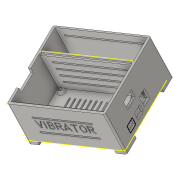
# Autodesk Inventor part: ARDUINO_DUE_CASE_BOTTOM
Saved by Autodesk Inventor 2016 (Build 200138000, 138)
## iProperties
Created: 2015-05-21
Part Number: ARDUINO_DUE_CASE_BOTTOM
Material: Generic
Document SubType Name: Modeling
Designer: Admin
Density: 1 g/cm^3
Appearance: Default
Author: Admin
Autodesk Inventor part; units mm, degrees
ref_plane "YZ Plane" through (0, 0, 0) normal (1, 0, 0) x (0, 1, 0)
ref_plane "XZ Plane" through (0, 0, 0) normal (0, 1, 0) x (-1, 0, 0)
ref_plane "XY Plane" through (0, 0, 0) normal (0, 0, 1) x (1, 0, 0)
sketch "Skizze1" plane through (0, 0, 0) normal (0, 1, 0) x (-1, 0, 0)
  line L0 (0, 0) -> (110, 0)
  line L1 (110, 0) -> (110, 88)
  line L2 (110, 88) -> (0, 88)
  line L3 (0, 88) -> (0, 0)
  dimension "d0" = 110
  dimension "d1" = 88
  constraints: 8 end point, 2 parallel, 1 horizontal, 1 perpendicular
  measures "d0" distance of L2.end L1.end
  measures "d1" distance of L1.end L0.end
extrude "Extrusion1" add sketch "Skizze1" along normal blind 50
sketch "Skizze2" plane through (0, 50, 0) normal (0, 1, 0) x (1, 0, 0)
  line L0 (-3, -5) -> (-107, -5)
  line L1 (-107, -5) -> (-107, -63)
  line L2 (-107, -63) -> (-3, -63)
  line L3 (-3, -63) -> (-3, -5)
  point P0 (0, 0)
  dimension "d4" = 104
  dimension "d5" = 58
  constraints: 8 end point, 2 parallel, 1 horizontal, 1 perpendicular
  measures "d4" distance of L2.end L1.end
  measures "d5" distance of L1.end L0.end
extrude "Extrusion2" cut sketch "Skizze2" against normal blind 47
sketch "Skizze3" plane through (0, 50, 0) normal (0, 1, 0) x (1, 0, 0)
  point P0 (0, 0)
sketch "Skizze6" plane through (0, 3, 0) normal (0, 1, 0) x (1, 0, 0)
  circle A0 centre (-91, -9.5) radius 4.5
  point P0 (0, 0)
  dimension "d16" = 9
  constraints: 1 centre point
  measures "d16" diameter of A0
extrude "Extrusion5" add sketch "Skizze6" along normal blind 4 draft -30
sketch "Skizze7" plane through (0, 3, 0) normal (0, 1, 0) x (1, 0, 0)
  circle A0 centre (-91, -58.5) radius 4.5
  point P0 (0, 0)
  dimension "d19" = 9
  constraints: 1 centre point
  measures "d19" diameter of A0
extrude "Extrusion6" add sketch "Skizze7" along normal blind 4 draft -30
sketch "Skizze8" plane through (-91, 7, 9.5) normal (0, 1, 0) x (1, 0, 0)
  point P0 (91, 9.5)
sketch "Skizze9" plane through (0, 3, 0) normal (0, 1, 0) x (1, 0, 0)
  circle A0 centre (-15.5, -9.5) radius 4.5
  point P0 (0, 0)
  dimension "d22" = 9
  constraints: 1 centre point
  measures "d22" diameter of A0
extrude "Extrusion7" add sketch "Skizze9" along normal blind 4 draft -30
sketch "Skizze10" plane through (0, 3, 0) normal (0, 1, 0) x (1, 0, 0)
  circle A0 centre (-9.5, -58.5) radius 4.5
  point P0 (0, 0)
  dimension "d25" = 9
  constraints: 1 centre point
  measures "d25" diameter of A0
extrude "Extrusion8" add sketch "Skizze10" along normal blind 4 draft -30
sketch "Skizze12" plane through (0, 50, 0) normal (0, 1, 0) x (1, 0, 0)
  line L0 (-3, -5) -> (-3, -63) projected
  line L1 (-3, -5) -> (-107, -5)
  line L2 (-107, -5) -> (-107, -3)
  line L3 (-107, -3) -> (-3, -3)
  line L4 (-3, -3) -> (-3, -5)
  point P0 (0, 0)
  dimension "d32" = 2
  constraints: 8 end point, 2 parallel, 1 horizontal, 1 perpendicular
  measures "d32" distance of L1.end L2.end
extrude "Extrusion10" cut sketch "Skizze12" against normal blind 2
sketch "Skizze13" plane through (0, 3, 0) normal (0, 1, 0) x (1, 0, 0)
  point P0 (0, 0)
sketch "Skizze14" plane through (0, 3, 0) normal (0, 1, 0) x (1, 0, 0)
  point P0 (0, 0)
sketch "Skizze15" plane through (-91, 7, 58.5) normal (0, 1, 0) x (1, 0, 0)
  circle A0 centre (0, 0) radius 1.25
  point P0 (91, 58.5)
  dimension "d35" = 2.5
  constraints: 1 centre point
  measures "d35" diameter of A0
extrude "Extrusion11" cut sketch "Skizze15" against normal blind 10
sketch "Skizze16" plane through (-91, 7, 9.5) normal (0, 1, 0) x (1, 0, 0)
  circle A0 centre (0, 0) radius 1.25
  point P0 (91, 9.5)
  dimension "d38" = 2.5
  constraints: 1 centre point
  measures "d38" diameter of A0
extrude "Extrusion12" cut sketch "Skizze16" against normal blind 10
sketch "Skizze17" plane through (-15.5, 7, 9.5) normal (0, 1, 0) x (1, 0, 0)
  circle A0 centre (0, 0) radius 1.25
  point P0 (15.5, 9.5)
  dimension "d41" = 2.5
  constraints: 1 centre point
  measures "d41" diameter of A0
extrude "Extrusion13" cut sketch "Skizze17" against normal blind 10
sketch "Skizze18" plane through (-9.5, 7, 58.5) normal (0, 1, 0) x (1, 0, 0)
  circle A0 centre (0, 0) radius 1.25
  point P0 (9.5, 58.5)
  dimension "d44" = 2.5
  constraints: 1 centre point
  measures "d44" diameter of A0
extrude "Extrusion14" cut sketch "Skizze18" against normal blind 10
sketch "Skizze29" plane through (0, 0, 0) normal (0, 0, -1) x (-1, 0, 0)
  line L0 (110, 50) -> (0, 50) construction
  line L1 (110, 0) -> (0, 0) construction
  line L2 (0, 50) -> (110, 0) construction
  line L3 (110, 50) -> (0, 0) construction
  line L4 (21.7553, 30.2834) -> (88.2914, 30.2834) construction
  line L5 (88.2914, 30.2834) -> (88.2914, 19.7381) construction
  line L6 (88.2914, 19.7381) -> (21.7553, 19.7381) construction
  line L7 (21.7553, 19.7381) -> (21.7553, 30.2834) construction
  line L8 (29.1209, 29.4232) -> (26.6631, 20.7135)
  spline S0 degree 2 poles (26.6631, 20.7135) (26.5172, 20.1913) (25.8951, 20.1913) knots 0 0 0 1 1 1
  spline S1 degree 2 poles (25.8951, 20.1913) (25.2653, 20.1913) (25.104, 20.6982) knots 0 0 0 1 1 1
  line L9 (25.104, 20.6982) -> (22.3467, 29.4078)
  spline S2 degree 2 poles (22.3467, 29.4078) (22.316, 29.5231) (22.316, 29.6306) knots 0 0 0 1 1 1
  spline S3 degree 2 poles (22.316, 29.6306) (22.316, 29.8764) (22.677, 30.2066) (22.9227, 30.2066) knots 0 0 0 1 2 2 2
  spline S4 degree 2 poles (22.9227, 30.2066) (23.3298, 30.2066) (23.4604, 29.7842) knots 0 0 0 1 1 1
  line L10 (23.4604, 29.7842) -> (25.8874, 22.3264)
  line L11 (25.8874, 22.3264) -> (27.9919, 29.7688)
  spline S5 degree 2 poles (27.9919, 29.7688) (28.1071, 30.2066) (28.5141, 30.2066) knots 0 0 0 1 1 1
  spline S6 degree 2 poles (28.5141, 30.2066) (28.7599, 30.2066) (29.1516, 29.8687) (29.1516, 29.5999) knots 0 0 0 1 2 2 2
  spline S7 degree 2 poles (29.1516, 29.5999) (29.1516, 29.5154) (29.1209, 29.4232) knots 0 0 0 1 1 1
  spline S8 degree 2 poles (32.5771, 20.8441) (32.5771, 20.222) (31.9857, 20.222) knots 0 0 0 1 1 1
  spline S9 degree 2 poles (31.9857, 20.222) (31.3866, 20.222) (31.3866, 20.8441) knots 0 0 0 1 1 1
  line L12 (31.3866, 20.8441) -> (31.3866, 29.5845)
  spline S10 degree 2 poles (31.3866, 29.5845) (31.3866, 30.1913) (31.9857, 30.1913) knots 0 0 0 1 1 1
  spline S11 degree 2 poles (31.9857, 30.1913) (32.5771, 30.1913) (32.5771, 29.5845) knots 0 0 0 1 1 1
  line L13 (32.5771, 29.5845) -> (32.5771, 20.8441)
  spline S12 degree 2 poles (41.8552, 23.1252) (41.8552, 20.3525) (38.7599, 20.3525) knots 0 0 0 1 1 1
  line L14 (38.7599, 20.3525) -> (35.4266, 20.3525)
  line L15 (35.4266, 20.3525) -> (35.4266, 30.2066)
  line L16 (35.4266, 30.2066) -> (38.6293, 30.2066)
  spline S13 degree 2 poles (38.6293, 30.2066) (40.081, 30.2066) (40.9258, 29.4539) knots 0 0 0 1 1 1
  spline S14 degree 2 poles (40.9258, 29.4539) (41.7246, 28.7089) (41.7246, 27.457) knots 0 0 0 1 1 1
  spline S15 degree 2 poles (41.7246, 27.457) (41.7246, 26.2281) (40.7184, 25.3525) knots 0 0 0 1 1 1
  spline S16 degree 2 poles (40.7184, 25.3525) (41.8552, 24.7151) (41.8552, 23.1252) knots 0 0 0 1 1 1
  spline S17 degree 2 poles (40.68, 23.1406) (40.68, 24.7688) (38.6831, 24.7688) knots 0 0 0 1 1 1
  line L17 (38.6831, 24.7688) -> (36.6017, 24.7688)
  line L18 (36.6017, 24.7688) -> (36.6017, 21.5737)
  line L19 (36.6017, 21.5737) -> (38.7599, 21.5737)
  spline S18 degree 2 poles (38.7599, 21.5737) (40.68, 21.5737) (40.68, 23.1406) knots 0 0 0 1 1 1
  spline S19 degree 2 poles (40.5495, 27.4724) (40.5495, 28.202) (39.5126, 28.9854) (38.6293, 28.9854) knots 0 0 0 1 2 2 2
  line L20 (38.6293, 28.9854) -> (36.6017, 28.9854)
  line L21 (36.6017, 28.9854) -> (36.6017, 25.99)
  line L22 (36.6017, 25.99) -> (38.7753, 25.99)
  spline S20 degree 2 poles (38.7753, 25.99) (40.5495, 25.99) (40.5495, 27.4724) knots 0 0 0 1 1 1
  spline S21 degree 2 poles (51.041, 27.3188) (51.041, 25.8057) (50.0502, 25.0453) knots 0 0 0 1 1 1
  spline S22 degree 2 poles (50.0502, 25.0453) (49.3974, 24.5538) (48.7446, 24.5538) knots 0 0 0 1 1 1
  line L23 (48.7446, 24.5538) -> (48.5986, 24.5461)
  line L24 (48.5986, 24.5461) -> (50.9258, 21.2128)
  spline S23 degree 2 poles (50.9258, 21.2128) (51.041, 21.0361) (51.041, 20.8441) knots 0 0 0 1 1 1
  spline S24 degree 2 poles (51.041, 20.8441) (51.041, 20.5983) (50.6647, 20.222) (50.4343, 20.222) knots 0 0 0 1 2 2 2
  spline S25 degree 2 poles (50.4343, 20.222) (50.1578, 20.222) (49.9811, 20.4831) knots 0 0 0 1 1 1
  line L25 (49.9811, 20.4831) -> (47.1163, 24.5538)
  line L26 (47.1163, 24.5538) -> (45.2115, 24.5538)
  line L27 (45.2115, 24.5538) -> (45.2115, 20.8441)
  spline S26 degree 2 poles (45.2115, 20.8441) (45.2115, 20.222) (44.6201, 20.222) knots 0 0 0 1 1 1
  spline S27 degree 2 poles (44.6201, 20.222) (44.0211, 20.222) (44.0211, 20.8441) knots 0 0 0 1 1 1
  line L28 (44.0211, 20.8441) -> (44.0211, 30.1836)
  line L29 (44.0211, 30.1836) -> (48.2223, 30.1836)
  spline S28 degree 2 poles (48.2223, 30.1836) (49.3667, 30.1836) (50.1808, 29.4386) knots 0 0 0 1 1 1
  spline S29 degree 2 poles (50.1808, 29.4386) (51.041, 28.6244) (51.041, 27.3188) knots 0 0 0 1 1 1
  spline S30 degree 2 poles (49.8659, 27.3188) (49.8659, 28.0868) (49.3744, 28.5553) knots 0 0 0 1 1 1
  spline S31 degree 2 poles (49.3744, 28.5553) (48.9058, 28.9777) (48.2223, 28.9777) knots 0 0 0 1 1 1
  line L30 (48.2223, 28.9777) -> (45.2115, 28.9777)
  line L31 (45.2115, 28.9777) -> (45.2115, 25.775)
  line L32 (45.2115, 25.775) -> (48.7446, 25.775)
  spline S32 degree 2 poles (48.7446, 25.775) (49.0671, 25.775) (49.3974, 26.0822) knots 0 0 0 1 1 1
  spline S33 degree 2 poles (49.3974, 26.0822) (49.8659, 26.5046) (49.8659, 27.3188) knots 0 0 0 1 1 1
  spline S34 degree 2 poles (60.5802, 21.0207) (60.6186, 20.8902) (60.6186, 20.775) knots 0 0 0 1 1 1
  spline S35 degree 2 poles (60.6186, 20.775) (60.6186, 20.5292) (60.2422, 20.2066) (60.0118, 20.2066) knots 0 0 0 1 2 2 2
  spline S36 degree 2 poles (60.0118, 20.2066) (59.5971, 20.2066) (59.4512, 20.583) knots 0 0 0 1 1 1
  line L33 (59.4512, 20.583) -> (58.8751, 22.0653)
  line L34 (58.8751, 22.0653) -> (54.1209, 22.0653)
  line L35 (54.1209, 22.0653) -> (53.5525, 20.583)
  spline S37 degree 2 poles (53.5525, 20.583) (53.4066, 20.2066) (53.0149, 20.2066) knots 0 0 0 1 1 1
  spline S38 degree 2 poles (53.0149, 20.2066) (52.7691, 20.2066) (52.3928, 20.5369) (52.3928, 20.775) knots 0 0 0 1 2 2 2
  spline S39 degree 2 poles (52.3928, 20.775) (52.3928, 20.8902) (52.4389, 21.0207) knots 0 0 0 1 1 1
  line L36 (52.4389, 21.0207) -> (55.7184, 29.8149)
  spline S40 degree 2 poles (55.7184, 29.8149) (55.8951, 30.2834) (56.4327, 30.2834) knots 0 0 0 1 1 1
  spline S41 degree 2 poles (56.4327, 30.2834) (56.9857, 30.2834) (57.1624, 29.8149) knots 0 0 0 1 1 1
  line L37 (57.1624, 29.8149) -> (60.5802, 21.0207)
  line L38 (58.422, 23.2865) -> (56.4327, 28.371)
  line L39 (56.4327, 28.371) -> (54.5817, 23.2865)
  line L40 (54.5817, 23.2865) -> (58.422, 23.2865)
  line L41 (68.7522, 28.9086) -> (66.1793, 28.9086)
  line L42 (66.1793, 28.9086) -> (66.1793, 20.3909)
  spline S42 degree 2 poles (66.1793, 20.3909) (66.1793, 19.7381) (65.5571, 19.7381) knots 0 0 0 1 1 1
  spline S43 degree 2 poles (65.5571, 19.7381) (64.9273, 19.7381) (64.9273, 20.3909) knots 0 0 0 1 1 1
  line L43 (64.9273, 20.3909) -> (64.9273, 28.9086)
  line L44 (64.9273, 28.9086) -> (62.3544, 28.9086)
  spline S44 degree 2 poles (62.3544, 28.9086) (61.7169, 28.9086) (61.7169, 29.5538) knots 0 0 0 1 1 1
  spline S45 degree 2 poles (61.7169, 29.5538) (61.7169, 30.1913) (62.3544, 30.1913) knots 0 0 0 1 1 1
  line L45 (62.3544, 30.1913) -> (68.7522, 30.1913)
  spline S46 degree 2 poles (68.7522, 30.1913) (69.3974, 30.1913) (69.3974, 29.5538) knots 0 0 0 1 1 1
  spline S47 degree 2 poles (69.3974, 29.5538) (69.3974, 28.9086) (68.7522, 28.9086) knots 0 0 0 1 1 1
  spline S48 degree 2 poles (78.4604, 25.1605) (78.4604, 23.1406) (77.485, 21.7043) knots 0 0 0 1 1 1
  spline S49 degree 2 poles (77.485, 21.7043) (76.425, 20.1452) (74.7507, 20.1452) knots 0 0 0 1 1 1
  spline S50 degree 2 poles (74.7507, 20.1452) (73.084, 20.1452) (72.0088, 21.7043) knots 0 0 0 1 1 1
  spline S51 degree 2 poles (72.0088, 21.7043) (70.9873, 23.1559) (70.9873, 25.1605) knots 0 0 0 1 1 1
  spline S52 degree 2 poles (70.9873, 25.1605) (70.9873, 27.1882) (71.9473, 28.6705) knots 0 0 0 1 1 1
  spline S53 degree 2 poles (71.9473, 28.6705) (72.9765, 30.2834) (74.5894, 30.2834) knots 0 0 0 1 1 1
  spline S54 degree 2 poles (74.5894, 30.2834) (76.3252, 30.2834) (77.4389, 28.6705) knots 0 0 0 1 1 1
  spline S55 degree 2 poles (77.4389, 28.6705) (78.4604, 27.1882) (78.4604, 25.1605) knots 0 0 0 1 1 1
  spline S56 degree 2 poles (77.2699, 25.1605) (77.2699, 26.7197) (76.6171, 27.8257) knots 0 0 0 1 1 1
  spline S57 degree 2 poles (76.6171, 27.8257) (75.8567, 29.0622) (74.5894, 29.0622) knots 0 0 0 1 1 1
  spline S58 degree 2 poles (74.5894, 29.0622) (73.4143, 29.0622) (72.7615, 27.8257) knots 0 0 0 1 1 1
  spline S59 degree 2 poles (72.7615, 27.8257) (72.1777, 26.7504) (72.1777, 25.1605) knots 0 0 0 1 1 1
  spline S60 degree 2 poles (72.1777, 25.1605) (72.1777, 23.6244) (72.8152, 22.5568) knots 0 0 0 1 1 1
  spline S61 degree 2 poles (72.8152, 22.5568) (73.5295, 21.3664) (74.7507, 21.3664) knots 0 0 0 1 1 1
  spline S62 degree 2 poles (74.7507, 21.3664) (75.9719, 21.3664) (76.6708, 22.5568) knots 0 0 0 1 1 1
  spline S63 degree 2 poles (76.6708, 22.5568) (77.2699, 23.6091) (77.2699, 25.1605) knots 0 0 0 1 1 1
  spline S64 degree 2 poles (87.2929, 27.3188) (87.2929, 25.8057) (86.3022, 25.0453) knots 0 0 0 1 1 1
  spline S65 degree 2 poles (86.3022, 25.0453) (85.6493, 24.5538) (84.9965, 24.5538) knots 0 0 0 1 1 1
  line L46 (84.9965, 24.5538) -> (84.8505, 24.5461)
  line L47 (84.8505, 24.5461) -> (87.1777, 21.2128)
  spline S66 degree 2 poles (87.1777, 21.2128) (87.2929, 21.0361) (87.2929, 20.8441) knots 0 0 0 1 1 1
  spline S67 degree 2 poles (87.2929, 20.8441) (87.2929, 20.5983) (86.9166, 20.222) (86.6862, 20.222) knots 0 0 0 1 2 2 2
  spline S68 degree 2 poles (86.6862, 20.222) (86.4097, 20.222) (86.233, 20.4831) knots 0 0 0 1 1 1
  line L48 (86.233, 20.4831) -> (83.3682, 24.5538)
  line L49 (83.3682, 24.5538) -> (81.4634, 24.5538)
  line L50 (81.4634, 24.5538) -> (81.4634, 20.8441)
  spline S69 degree 2 poles (81.4634, 20.8441) (81.4634, 20.222) (80.872, 20.222) knots 0 0 0 1 1 1
  spline S70 degree 2 poles (80.872, 20.222) (80.273, 20.222) (80.273, 20.8441) knots 0 0 0 1 1 1
  line L51 (80.273, 20.8441) -> (80.273, 30.1836)
  line L52 (80.273, 30.1836) -> (84.4742, 30.1836)
  spline S71 degree 2 poles (84.4742, 30.1836) (85.6186, 30.1836) (86.4327, 29.4386) knots 0 0 0 1 1 1
  spline S72 degree 2 poles (86.4327, 29.4386) (87.2929, 28.6244) (87.2929, 27.3188) knots 0 0 0 1 1 1
  spline S73 degree 2 poles (86.1178, 27.3188) (86.1178, 28.0868) (85.6263, 28.5553) knots 0 0 0 1 1 1
  spline S74 degree 2 poles (85.6263, 28.5553) (85.1578, 28.9777) (84.4742, 28.9777) knots 0 0 0 1 1 1
  line L53 (84.4742, 28.9777) -> (81.4634, 28.9777)
  line L54 (81.4634, 28.9777) -> (81.4634, 25.775)
  line L55 (81.4634, 25.775) -> (84.9965, 25.775)
  spline S75 degree 2 poles (84.9965, 25.775) (85.3191, 25.775) (85.6493, 26.0822) knots 0 0 0 1 1 1
  spline S76 degree 2 poles (85.6493, 26.0822) (86.1178, 26.5046) (86.1178, 27.3188) knots 0 0 0 1 1 1
  constraints: 4 end point, 2 other
extrude "Extrusion25" cut sketch "Skizze29" against normal blind 1
fillet "Rundung1" radius 2 1 edges at (-110, 25, 0)
fillet "Rundung3" radius 2 1 edges at (0, 25, 0)
sketch "Skizze30" plane through (0, 0, 0) normal (0, -1, 0) x (1, 0, 0)
  circle A0 centre (-15.5, 9.5) radius 1.25 projected
  circle A1 centre (-15.5, 9.5) radius 6
  point P0 (0, 0)
  dimension "d89" = 12
  constraints: 1 centre point, 1 coincident
  measures "d89" diameter of A1
extrude "Extrusion26" add sketch "Skizze30" along normal blind 5 draft -20
sketch "Skizze31" plane through (0, 0, 0) normal (0, -1, 0) x (1, 0, 0)
  circle A0 centre (-91, 9.5) radius 1.25 projected
  circle A1 centre (-91, 9.5) radius 6
  point P0 (0, 0)
  dimension "d92" = 12
  constraints: 1 centre point, 1 coincident
  measures "d92" diameter of A1
extrude "Extrusion27" add sketch "Skizze31" along normal blind 5 draft -20
sketch "Skizze32" plane through (0, 0, 0) normal (0, -1, 0) x (1, 0, 0)
  circle A0 centre (-91, 9.5) radius 6 projected
  circle A1 centre (-15.5, 9.5) radius 6 projected
  arc A2 (-2, 0) -> (0, 2) centre (-2, 2) ccw projected
  line L0 (0, 88) -> (0, 2) projected
  line L1 (-110, 88) -> (0, 88) projected
  line L2 (-110, 2) -> (-110, 88) projected
  arc A3 (-110, 2) -> (-108, 0) centre (-108, 2) ccw projected
  line L3 (-2, 0) -> (-108, 0) projected
  circle A4 centre (-9.5, 58.5) radius 1.25 projected
  circle A5 centre (-91, 58.5) radius 1.25 projected
  point P0 (0, 0)
sketch "Skizze33" plane through (0, 0, 0) normal (0, -1, 0) x (1, 0, 0)
  circle A0 centre (-9.5, 58.5) radius 1.25 projected
  circle A1 centre (-9.5, 58.5) radius 6
  point P0 (0, 0)
  dimension "d95" = 12
  constraints: 1 centre point, 1 coincident
  measures "d95" diameter of A1
extrude "Extrusion28" add sketch "Skizze33" along normal blind 5 draft -20
sketch "Skizze34" plane through (0, 0, 0) normal (0, -1, 0) x (1, 0, 0)
  circle A0 centre (-91, 58.5) radius 1.25 projected
  circle A1 centre (-91, 58.5) radius 6
  point P0 (0, 0)
  dimension "d98" = 12
  constraints: 1 centre point, 1 coincident
  measures "d98" diameter of A1
extrude "Extrusion29" add sketch "Skizze34" along normal blind 5 draft -20
sketch "Skizze35" plane through (-15.5, -5, 9.5) normal (0, -1, 0) x (1, 0, 0)
  circle A0 centre (0, 0) radius 3.0699 projected
  circle A1 centre (0, 0) radius 3
  point P0 (15.5, -9.5)
  dimension "d101" = 6
  constraints: 1 centre point, 1 coincident
  measures "d101" diameter of A1
extrude "Extrusion30" cut sketch "Skizze35" against normal blind 5 contours A1
sketch "Skizze36" plane through (-91, -5, 9.5) normal (0, -1, 0) x (1, 0, 0)
  circle A0 centre (0, 0) radius 1.25 projected
  circle A1 centre (0, 0) radius 3
  point P0 (91, -9.5)
  dimension "d104" = 6
  constraints: 1 centre point, 1 coincident
  measures "d104" diameter of A1
extrude "Extrusion31" cut sketch "Skizze36" against normal blind 5
sketch "Skizze37" plane through (-91, -5, 58.5) normal (0, -1, 0) x (1, 0, 0)
  circle A0 centre (0, 0) radius 3
  point P0 (91, -58.5)
  dimension "d107" = 6
  constraints: 1 centre point
  measures "d107" diameter of A0
extrude "Extrusion32" cut sketch "Skizze37" against normal blind 5
sketch "Skizze38" plane through (-9.5, -5, 58.5) normal (0, -1, 0) x (1, 0, 0)
  circle A0 centre (0, 0) radius 3
  point P0 (9.5, -58.5)
  dimension "d110" = 6
  constraints: 1 centre point
  measures "d110" diameter of A0
extrude "Extrusion33" cut sketch "Skizze38" against normal blind 5
sketch "Skizze39" plane through (-108, 0, 0) normal (0, 0, -1) x (-1, 0, 0)
  line L0 (-86, 34) -> (-20, 34) construction
  line L1 (2, 0) -> (2, 50) projected
  line L2 (-86, 33) -> (-20, 33)
  line L3 (-20, 35) -> (-86, 35)
  arc A0 (-86, 35) -> (-86, 33) centre (-86, 34) ccw
  arc A1 (-20, 33) -> (-20, 35) centre (-20, 34) ccw
  point P0 (-108, 0)
  point P1 (-53, 34)
  dimension "d113" = 66
  dimension "d114" = 2
  constraints: 8 end point, 4 point on circle, 4 tangent, 2 centre point, 1 midpoint, 1 parallel, 1 perpendicular
  measures "d113" distance of L0.start L0.end
  measures "d114" diameter of A1
extrude "Extrusion34" cut sketch "Skizze39" against normal blind 5
sketch "Skizze40" plane through (-108, 0, 0) normal (0, 0, -1) x (-1, 0, 0)
  line L0 (-86, 14) -> (-20, 14) construction
  line L1 (-86, 13) -> (-20, 13)
  line L2 (-20, 15) -> (-86, 15)
  arc A0 (-86, 15) -> (-86, 13) centre (-86, 14) ccw
  arc A1 (-20, 13) -> (-20, 15) centre (-20, 14) ccw
  point P0 (-108, 0)
  point P1 (-53, 14)
  dimension "d117" = 2
  constraints: 8 end point, 4 point on circle, 4 tangent, 2 centre point, 1 horizontal, 1 midpoint, 1 parallel
  measures "d117" diameter of A1
extrude "Extrusion35" cut sketch "Skizze40" against normal blind 5
sketch "Skizze43" plane through (-91, 7, 58.5) normal (0, 1, 0) x (1, 0, 0)
  circle A0 centre (0, 0) radius 1.25 projected
  circle A1 centre (0, 0) radius 2.1906 projected
  circle A2 centre (0, 0) radius 1.75
  point P0 (91, 58.5)
  dimension "d126" = 3.5
  constraints: 1 centre point, 1 coincident
  measures "d126" diameter of A2
extrude "Extrusion38" cut sketch "Skizze43" against normal blind 10 contours A2
sketch "Skizze44" plane through (-91, 7, 9.5) normal (0, 1, 0) x (1, 0, 0)
  circle A0 centre (0, 0) radius 1.25 projected
  circle A1 centre (0, 0) radius 2.1906 projected
  circle A2 centre (0, 0) radius 1.75
  point P0 (91, 9.5)
  dimension "d129" = 3.5
  constraints: 1 centre point, 1 coincident
  measures "d129" diameter of A2
extrude "Extrusion39" cut sketch "Skizze44" against normal blind 10 contours A2
sketch "Skizze45" plane through (-15.5, 7, 9.5) normal (0, 1, 0) x (1, 0, 0)
  circle A0 centre (0, 0) radius 1.25 projected
  circle A1 centre (0, 0) radius 2.1906 projected
  circle A2 centre (0, 0) radius 1.75
  point P0 (15.5, 9.5)
  dimension "d132" = 3.5
  constraints: 1 centre point, 1 coincident
  measures "d132" diameter of A2
extrude "Extrusion40" cut sketch "Skizze45" against normal blind 10 contours A2
sketch "Skizze46" plane through (-9.5, 7, 58.5) normal (0, 1, 0) x (1, 0, 0)
  circle A0 centre (0, 0) radius 1.25 projected
  circle A1 centre (0, 0) radius 2.1906 projected
  circle A2 centre (0, 0) radius 1.75
  point P0 (9.5, 58.5)
  dimension "d135" = 3.5
  constraints: 1 centre point, 1 coincident
  measures "d135" diameter of A2
extrude "Extrusion41" cut sketch "Skizze46" against normal blind 10 contours A2
sketch "Skizze49" plane through (-110, 0, 88) normal (0, 0, 1) x (1, 0, 0)
  line L0 (110, 0) -> (108, 0) projected
  line L1 (110, 0) -> (0, 0)
  line L2 (0, 0) -> (0, 50)
  line L3 (0, 50) -> (110, 50)
  line L4 (110, 50) -> (110, 0)
  constraints: 8 end point, 2 parallel, 1 horizontal, 1 perpendicular
extrude "Extrusion44" add sketch "Skizze49" along normal blind 10
sketch "Skizze50" plane through (0, 50, 0) normal (0, 1, 0) x (1, 0, 0)
  line L0 (-4, -67) -> (-106, -67)
  line L1 (-106, -67) -> (-106, -94)
  line L2 (-106, -94) -> (-4, -94)
  line L3 (-4, -94) -> (-4, -67)
  point P0 (0, 0)
  constraints: 8 end point, 2 parallel, 1 horizontal, 1 perpendicular
extrude "Extrusion45" cut sketch "Skizze50" against normal blind 48
fillet "Rundung5" radius 2 1 edges at (-110, 25, 98)
fillet "Rundung6" radius 2 1 edges at (0, 25, 98)
sketch "Skizze53" plane through (0, 50, 0) normal (0, 1, 0) x (1, 0, 0)
  line L0 (-3, -63) -> (-9.5, -63) projected
  line L1 (-4, -63) -> (-106, -63)
  line L2 (-106, -63) -> (-106, -65)
  line L3 (-106, -65) -> (-4, -65)
  line L4 (-4, -65) -> (-4, -63)
  point P0 (0, 0)
  constraints: 8 end point, 2 parallel, 1 horizontal, 1 perpendicular, 1 point on line
extrude "Extrusion48" cut sketch "Skizze53" against normal blind 2
sketch "Skizze54" plane through (-3, 3, 63) normal (-1, 0, 0) x (0, 0, 1)
  line L0 (-61, 47) -> (33, 47) projected
  line L1 (-43, 41) -> (-18, 41)
  line L2 (-18, 41) -> (-18, 47)
  line L3 (-18, 47) -> (-43, 47)
  line L4 (-43, 47) -> (-43, 41)
  point P0 (-63, -3)
  constraints: 8 end point, 2 parallel, 1 horizontal, 1 perpendicular, 1 point on line
extrude "Extrusion49" cut sketch "Skizze54" against normal blind 10
sketch "Skizze55" plane through (-107, 3, 63) normal (1, 0, 0) x (0, 0, -1)
  line L0 (15, 5) -> (4, 5)
  line L1 (4, 5) -> (4, 18)
  line L2 (4, 18) -> (15, 18)
  line L3 (15, 18) -> (15, 5)
  point P0 (63, -3)
  constraints: 8 end point, 2 parallel, 1 horizontal, 1 perpendicular
extrude "Extrusion50" cut sketch "Skizze55" against normal blind 10
sketch "Skizze56" plane through (-110, 0, 2) normal (-1, 0, 0) x (0, 0, 1)
  line L0 (42, 6) -> (31, 6)
  line L1 (31, 6) -> (31, 15)
  line L2 (31, 15) -> (42, 15)
  line L3 (42, 15) -> (42, 6)
  point P0 (-2, 0)
  constraints: 8 end point, 2 parallel, 1 horizontal, 1 perpendicular
extrude "Extrusion51" cut sketch "Skizze56" against normal blind 10
sketch "Skizze57" plane through (-110, 0, 2) normal (-1, 0, 0) x (0, 0, 1)
  line L0 (26, 6) -> (15, 6)
  line L1 (15, 6) -> (15, 15)
  line L2 (15, 15) -> (26, 15)
  line L3 (26, 15) -> (26, 6)
  point P0 (-2, 0)
  constraints: 8 end point, 2 parallel, 1 horizontal, 1 perpendicular
extrude "Extrusion52" cut sketch "Skizze57" against normal blind 10
sketch "Skizze58" plane through (-110, 0, 98) normal (0, 0, 1) x (1, 0, 0)
  line L0 (108, 50) -> (108, 0) projected
  line L1 (10, 40) -> (100, 40) construction
  line L2 (10, 41) -> (100, 41)
  line L3 (100, 39) -> (10, 39)
  arc A0 (10, 41) -> (10, 39) centre (10, 40) ccw
  arc A1 (100, 39) -> (100, 41) centre (100, 40) ccw
  point P0 (110, 0)
  point P1 (55, 40)
  constraints: 8 end point, 4 point on circle, 4 tangent, 2 centre point, 1 midpoint, 1 parallel, 1 perpendicular
extrude "Extrusion53" cut sketch "Skizze58" against normal blind 10
sketch "Skizze59" plane through (-110, 0, 98) normal (0, 0, 1) x (1, 0, 0)
  line L0 (10, 10) -> (100, 10) construction
  line L1 (22, 13) -> (88, 13) projected
  line L2 (10, 11) -> (100, 11)
  line L3 (100, 9) -> (10, 9)
  arc A0 (10, 11) -> (10, 9) centre (10, 10) ccw
  arc A1 (100, 9) -> (100, 11) centre (100, 10) ccw
  point P0 (110, 0)
  point P1 (55, 10)
  constraints: 8 end point, 4 point on circle, 4 tangent, 2 centre point, 2 parallel, 1 midpoint
extrude "Extrusion54" cut sketch "Skizze59" against normal blind 10
sketch "Skizze60" plane through (-106, 50, 67) normal (0, 0, 1) x (1, 0, 0)
  line L0 (102, 0) -> (102, -48) projected
  line L1 (10, -10) -> (92, -10) construction
  line L2 (10, -9) -> (92, -9)
  line L3 (92, -11) -> (10, -11)
  arc A0 (10, -9) -> (10, -11) centre (10, -10) ccw
  arc A1 (92, -11) -> (92, -9) centre (92, -10) ccw
  line L4 (51.9213, -34) -> (51.9213, -42) construction
  line L5 (10, -19) -> (92, -19) construction
  line L6 (10, -18) -> (92, -18)
  line L7 (92, -20) -> (10, -20)
  arc A2 (10, -18) -> (10, -20) centre (10, -19) ccw
  arc A3 (92, -20) -> (92, -18) centre (92, -19) ccw
  line L8 (10, -28) -> (92, -28) construction
  line L9 (10, -27) -> (92, -27)
  line L10 (92, -29) -> (10, -29)
  arc A4 (10, -27) -> (10, -29) centre (10, -28) ccw
  arc A5 (92, -29) -> (92, -27) centre (92, -28) ccw
  line L11 (10, -37) -> (92, -37) construction
  line L12 (10, -36) -> (92, -36)
  line L13 (92, -38) -> (10, -38)
  arc A6 (10, -36) -> (10, -38) centre (10, -37) ccw
  arc A7 (92, -38) -> (92, -36) centre (92, -37) ccw
  point P0 (106, -50)
  point P1 (51, -10)
  point P2 (51, -19)
  point P3 (51, -28)
  point P4 (51, -37)
  dimension "d170" = 9
  constraints: 34 end point, 16 point on circle, 8 centre point, 4 tangent, 2 vertical, 1 midpoint, 1 parallel, 1 perpendicular, 36 other
  measures "d170" distance of L2.start L6.start
extrude "Extrusion55" cut sketch "Skizze60" against normal blind 10
sketch "Skizze61" plane through (0, 0, 0) normal (0, -1, 0) x (1, 0, 0)
  arc A0 (0, 96) -> (-2, 98) centre (-2, 96) ccw projected
  line L0 (0, 2) -> (0, 96) projected
  line L1 (-2, 98) -> (-108, 98) projected
  line L2 (0, 78) -> (-4, 78)
  line L3 (-4, 78) -> (-4, 98)
  line L4 (-4, 98) -> (0, 98)
  line L5 (0, 98) -> (0, 78)
  line L6 (-100, 98) -> (-10, 98) projected
  line L7 (-4, 94) -> (-106, 94) projected
  line L8 (-22, 98) -> (-4, 98)
  line L9 (-4, 98) -> (-4, 94)
  line L10 (-4, 94) -> (-22, 94)
  line L11 (-22, 94) -> (-22, 98)
  point P0 (0, 0)
  constraints: 16 end point, 4 parallel, 3 point on line, 2 horizontal, 2 perpendicular
extrude "Extrusion56" add sketch "Skizze61" along normal blind 5 contours L0 L2 L3 L1 A0 | L3 L7 L11 L1
sketch "Skizze62" plane through (0, 0, 0) normal (0, -1, 0) x (1, 0, 0)
  line L0 (-108, 98) -> (-22, 98) projected
  line L1 (-110, 98) -> (-88, 98)
  line L2 (-88, 98) -> (-88, 94)
  line L3 (-88, 94) -> (-110, 94)
  line L4 (-110, 94) -> (-110, 98)
  line L5 (-106, 94) -> (-106, 67) projected
  line L6 (-106, 78) -> (-110, 78)
  line L7 (-110, 78) -> (-110, 94)
  line L8 (-110, 94) -> (-106, 94)
  line L9 (-106, 94) -> (-106, 78)
  point P0 (0, 0)
  constraints: 16 end point, 4 parallel, 2 horizontal, 2 perpendicular, 2 point on line
extrude "Extrusion57" add sketch "Skizze62" along normal blind 5
fillet "Rundung7" radius 2 1 edges at (-110, -2.5, 98)
sketch "Skizze63" plane through (0, 0, 0) normal (0, -1, 0) x (1, 0, 0)
  line L0 (-2, 0) -> (-108, 0) projected
  arc A0 (-2, 0) -> (0, 2) centre (-2, 2) ccw projected
  line L1 (0, 2) -> (0, 78) projected
  line L2 (0, 20) -> (-4, 20)
  line L3 (-4, 20) -> (-4, 0)
  line L4 (-4, 0) -> (0, 0)
  line L5 (0, 0) -> (0, 20)
  line L6 (-12, 0) -> (-4, 0)
  line L7 (-4, 0) -> (-4, 4)
  line L8 (-4, 4) -> (-12, 4)
  line L9 (-12, 4) -> (-12, 0)
  constraints: 16 end point, 4 parallel, 2 horizontal, 2 perpendicular, 2 point on line
extrude "Extrusion58" add sketch "Skizze63" along normal blind 5 contours L0 L3 L2 L1 A0 | L0 L9 L8 L3
sketch "Skizze64" plane through (0, 0, 0) normal (0, -1, 0) x (1, 0, 0)
  line L0 (-110, 2) -> (-110, 78) projected
  arc A0 (-110, 2) -> (-108, 0) centre (-108, 2) ccw projected
  line L1 (-12, 4) -> (-4, 4) projected
  line L2 (-2, 0) -> (-108, 0) projected
  line L3 (-110, 20) -> (-106, 20)
  line L4 (-106, 20) -> (-106, 0)
  line L5 (-106, 0) -> (-110, 0)
  line L6 (-110, 0) -> (-110, 20)
  line L7 (-98, 4) -> (-106, 4)
  line L8 (-106, 4) -> (-106, 0)
  line L9 (-106, 0) -> (-98, 0)
  line L10 (-98, 0) -> (-98, 4)
  point P0 (0, 0)
  constraints: 16 end point, 4 parallel, 3 point on line, 2 horizontal, 2 perpendicular
extrude "Extrusion59" add sketch "Skizze64" along normal blind 5 contours L0 L3 L4 L2 A0 | L4 L7 L10 L2
sketch "Skizze65" plane through (-3, 3, 63) normal (0, 0, -1) x (-1, 0, 0)
  circle A0 centre (100, 4) radius 4
  point P0 (-3, -3)
  constraints: 1 centre point
extrude "Extrusion60" cut sketch "Skizze65" against normal blind 5
sketch "Skizze66" plane through (0, 3, 0) normal (0, 1, 0) x (1, 0, 0)
  line L0 (-22, -52) -> (-22, -16) construction
  line L1 (-21, -52) -> (-21, -16)
  line L2 (-23, -16) -> (-23, -52)
  arc A0 (-23, -52) -> (-21, -52) centre (-22, -52) ccw
  arc A1 (-21, -16) -> (-23, -16) centre (-22, -16) ccw
  line L3 (-37, -34) -> (-43.5613, -34) construction
  arc A2 (-27, -16) -> (-29, -16) centre (-28, -16) ccw
  line L4 (-28, -52) -> (-28, -16) construction
  line L5 (-27, -52) -> (-27, -16)
  arc A3 (-29, -52) -> (-27, -52) centre (-28, -52) ccw
  line L6 (-29, -16) -> (-29, -52)
  arc A4 (-33, -16) -> (-35, -16) centre (-34, -16) ccw
  line L7 (-34, -52) -> (-34, -16) construction
  line L8 (-33, -52) -> (-33, -16)
  arc A5 (-35, -52) -> (-33, -52) centre (-34, -52) ccw
  line L9 (-35, -16) -> (-35, -52)
  arc A6 (-39, -16) -> (-41, -16) centre (-40, -16) ccw
  line L10 (-40, -52) -> (-40, -16) construction
  line L11 (-39, -52) -> (-39, -16)
  arc A7 (-41, -52) -> (-39, -52) centre (-40, -52) ccw
  line L12 (-41, -16) -> (-41, -52)
  arc A8 (-45, -16) -> (-47, -16) centre (-46, -16) ccw
  line L13 (-46, -52) -> (-46, -16) construction
  line L14 (-45, -52) -> (-45, -16)
  arc A9 (-47, -52) -> (-45, -52) centre (-46, -52) ccw
  line L15 (-47, -16) -> (-47, -52)
  arc A10 (-51, -16) -> (-53, -16) centre (-52, -16) ccw
  line L16 (-52, -52) -> (-52, -16) construction
  line L17 (-51, -52) -> (-51, -16)
  arc A11 (-53, -52) -> (-51, -52) centre (-52, -52) ccw
  line L18 (-53, -16) -> (-53, -52)
  arc A12 (-57, -16) -> (-59, -16) centre (-58, -16) ccw
  line L19 (-58, -52) -> (-58, -16) construction
  line L20 (-57, -52) -> (-57, -16)
  arc A13 (-59, -52) -> (-57, -52) centre (-58, -52) ccw
  line L21 (-59, -16) -> (-59, -52)
  arc A14 (-63, -16) -> (-65, -16) centre (-64, -16) ccw
  line L22 (-64, -52) -> (-64, -16) construction
  line L23 (-63, -52) -> (-63, -16)
  arc A15 (-65, -52) -> (-63, -52) centre (-64, -52) ccw
  line L24 (-65, -16) -> (-65, -52)
  arc A16 (-69, -16) -> (-71, -16) centre (-70, -16) ccw
  line L25 (-70, -52) -> (-70, -16) construction
  line L26 (-69, -52) -> (-69, -16)
  arc A17 (-71, -52) -> (-69, -52) centre (-70, -52) ccw
  line L27 (-71, -16) -> (-71, -52)
  arc A18 (-75, -16) -> (-77, -16) centre (-76, -16) ccw
  line L28 (-76, -52) -> (-76, -16) construction
  line L29 (-75, -52) -> (-75, -16)
  arc A19 (-77, -52) -> (-75, -52) centre (-76, -52) ccw
  line L30 (-77, -16) -> (-77, -52)
  arc A20 (-81, -16) -> (-83, -16) centre (-82, -16) ccw
  line L31 (-82, -52) -> (-82, -16) construction
  line L32 (-81, -52) -> (-81, -16)
  arc A21 (-83, -52) -> (-81, -52) centre (-82, -52) ccw
  line L33 (-83, -16) -> (-83, -52)
  point P0 (0, 0)
  point P1 (-22, -34)
  point P2 (-28, -34)
  point P3 (-34, -34)
  point P4 (-40, -34)
  point P5 (-46, -34)
  point P6 (-52, -34)
  point P7 (-58, -34)
  point P8 (-64, -34)
  point P9 (-70, -34)
  point P10 (-76, -34)
  point P11 (-82, -34)
  dimension "d190" = 6
  constraints: 90 end point, 44 point on circle, 22 centre point, 4 tangent, 2 horizontal, 1 midpoint, 1 parallel, 1 vertical, 120 other
  measures "d190" distance of L2.start L6.start
extrude "Extrusion61" cut sketch "Skizze66" against normal blind 10
sketch "Skizze68" plane through (-4, 50, 94) normal (0, 0, -1) x (-1, 0, 0)
  arc A0 (96, -41) -> (96, -39) centre (96, -40) ccw projected
  line L0 (96, -41) -> (6, -41) projected
  arc A1 (6, -39) -> (6, -41) centre (6, -40) ccw projected
  line L1 (6, -39) -> (96, -39) projected
  arc A2 (96, -11) -> (96, -9) centre (96, -10) ccw projected
  line L2 (96, -11) -> (6, -11) projected
  arc A3 (6, -9) -> (6, -11) centre (6, -10) ccw projected
  line L3 (6, -9) -> (96, -9) projected
  line L4 (0, 0) -> (102, 0) projected
  line L5 (0, 0) -> (0, -48) projected
  line L6 (0, -48) -> (102, -48)
  line L7 (102, -48) -> (102, 0)
  line L8 (102, 0) -> (0, 0)
  line L9 (0, 0) -> (0, -48)
  point P0 (-4, -50)
  constraints: 8 end point, 2 parallel, 1 horizontal, 1 perpendicular
extrude "Extrusion63" cut sketch "Skizze68" against normal blind 2
sketch "Skizze69" plane through (-110, 50, 2) normal (-1, 0, 0) x (0, 0, 1)
  line L0 (26, -24) -> (42, -24)
  line L1 (42, -24) -> (42, -14)
  line L2 (42, -14) -> (26, -14)
  line L3 (26, -14) -> (26, -24)
  point P0 (-2, -50)
  constraints: 8 end point, 2 parallel, 1 horizontal, 1 perpendicular
extrude "Extrusion65" cut sketch "Skizze69" against normal blind 10
sketch "Skizze70" plane through (-106, 50, 67) normal (0, 0, 1) x (1, 0, 0)
  arc A0 (0, -45.6458) -> (0, -40.3542) centre (3, -43) ccw projected
  line L0 (0, -45.6458) -> (0, -48) projected
  line L1 (0, -48) -> (102, -48) projected
  line L2 (102, 0) -> (102, -48) projected
  line L3 (0, 0) -> (102, 0) projected
  line L4 (0, 0) -> (0, -40.3542) projected
  arc A1 (10, -36) -> (10, -38) centre (10, -37) ccw projected
  line L5 (10, -36) -> (92, -36) projected
  arc A2 (92, -38) -> (92, -36) centre (92, -37) ccw projected
  line L6 (92, -38) -> (10, -38) projected
  arc A3 (10, -18) -> (10, -20) centre (10, -19) ccw projected
  line L7 (10, -18) -> (92, -18) projected
  arc A4 (92, -20) -> (92, -18) centre (92, -19) ccw projected
  line L8 (92, -20) -> (10, -20) projected
  arc A5 (10, -9) -> (10, -11) centre (10, -10) ccw projected
  line L9 (10, -9) -> (92, -9) projected
  arc A6 (92, -11) -> (92, -9) centre (92, -10) ccw projected
  line L10 (92, -11) -> (10, -11) projected
  arc A7 (10, -27) -> (10, -29) centre (10, -28) ccw projected
  line L11 (10, -27) -> (92, -27) projected
  arc A8 (92, -29) -> (92, -27) centre (92, -28) ccw projected
  line L12 (92, -29) -> (10, -29) projected
  point P0 (106, -50)
sketch "Skizze71" plane through (-4, 2, 67) normal (-1, 0, 0) x (0, 0, 1)
  line L0 (0, 48) -> (29, 48)
  line L1 (29, 48) -> (29, 0)
  line L2 (29, 0) -> (0, 0)
  line L3 (0, 0) -> (0, 48)
  point P0 (-67, -2)
  constraints: 8 end point, 2 parallel, 1 horizontal, 1 perpendicular
extrude "Extrusion66" cut sketch "Skizze71" against normal blind 1
sketch "Skizze72" plane through (-106, 9.6458, 67) normal (1, 0, 0) x (0, 0, -1)
  line L0 (-1, 0) -> (0, 0) projected
  line L1 (0, 40.3542) -> (0, 0) projected
  line L2 (-29, 40.3542) -> (0, 40.3542) projected
  line L3 (0, -5.2915) -> (0, -7.6458) projected
  line L4 (0, -5.2915) -> (-1, -5.2915) projected
  line L5 (-1, -5.2915) -> (-1, 0) projected
  line L6 (-29, 40.3542) -> (-29, -14.6458) projected
  line L7 (0, -7.6458) -> (-29, -7.6458)
  line L8 (-29, -7.6458) -> (-29, 40.3542)
  line L9 (-29, 40.3542) -> (0, 40.3542)
  line L10 (0, 40.3542) -> (0, -7.6458)
  line L11 (-31, 40.3542) -> (-29, 40.3542) projected
  line L12 (0, -7.6458) -> (-29, -7.6458)
  line L13 (-29, -7.6458) -> (-29, 40.3542)
  line L14 (-29, 40.3542) -> (0, 40.3542)
  line L15 (0, 40.3542) -> (0, -7.6458)
  point P0 (67, -9.6458)
  constraints: 16 end point, 4 parallel, 2 horizontal, 2 perpendicular
extrude "Extrusion67" cut sketch "Skizze72" against normal blind 1 contours L5 L4 L3 L7 L6 L2 L1 L0
sketch "Skizze73" plane through (0, 0, 0) normal (0, -1, 0) x (1, 0, 0)
  line L0 (-106, 94) -> (-106, 78) projected
  line L1 (-9.5, 82) -> (-99, 82) construction
  line L2 (-9.5, 83) -> (-99, 83)
  line L3 (-99, 81) -> (-9.5, 81)
  arc A0 (-9.5, 81) -> (-9.5, 83) centre (-9.5, 82) ccw
  arc A1 (-99, 83) -> (-99, 81) centre (-99, 82) ccw
  point P0 (0, 0)
  point P1 (-54.25, 82)
  dimension "d209" = 2
  constraints: 8 end point, 4 point on circle, 4 tangent, 2 centre point, 1 midpoint, 1 parallel, 1 perpendicular
  measures "d209" diameter of A1
extrude "Extrusion68" cut sketch "Skizze73" against normal blind 5
